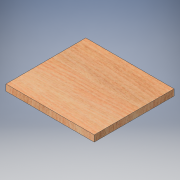
# Autodesk Inventor part: topPlate
Saved by Autodesk Inventor 2016 (Build 200138000, 138)
## iProperties
Created: 2015-09-21
Part Number: topPlate
Material: Generic
Document SubType Name: Modeling
Designer: xdlea
Density: 1 g/cm^3
Appearance: Birch - Natural Polished
Length: 10.500 in
Width: 8.000 in
Thickness: 0.750 in
RailHeight: 2.000 in
Author: xdlea
Autodesk Inventor part; units mm, degrees
ref_plane "YZ Plane" through (0, 0, 0) normal (1, 0, 0) x (0, 1, 0)
ref_plane "XZ Plane" through (0, 0, 0) normal (0, 1, 0) x (-1, 0, 0)
ref_plane "XY Plane" through (0, 0, 0) normal (0, 0, 1) x (1, 0, 0)
sketch "Sketch1" plane through (0, 0, 0) normal (0, 1, 0) x (-1, 0, 0)
  line L0 (133.35, 101.6) -> (-133.35, 101.6)
  line L1 (-133.35, 101.6) -> (-133.35, -101.6)
  line L2 (-133.35, -101.6) -> (133.35, -101.6)
  line L3 (133.35, -101.6) -> (133.35, 101.6)
  line L4 (133.35, 101.6) -> (-133.35, -101.6) construction
  line L5 (-133.35, 101.6) -> (133.35, -101.6) construction
  point P0 (0, 0)
  dimension "d0" = 266.7
  dimension "d1" = 203.2
  constraints: 12 end point, 2 midpoint, 2 parallel, 1 horizontal, 1 perpendicular
  measures "d0" distance of L0.start L0.end
  measures "d1" distance of L0.end L1.end
extrude "Extrusion1" add sketch "Sketch1" along normal blind 19.05
sketch "Sketch2" plane through (-133.35, 0, 101.6) normal (0, 0, 1) x (1, 0, 0)
  line L0 (0, 0) -> (266.7, 0) projected
  line L1 (266.7, 0) -> (266.7, 19.05) projected
  line L2 (0, 19.05) -> (266.7, 19.05) projected
  line L3 (0, 0) -> (0, 19.05) projected
  point P0 (133.35, 0)
extrude "Extrusion2" add sketch "Sketch2" along normal blind 38.1
equation "\"d0\" = Length"
equation "\"d1\" = Width"
equation "\"d2\" = Thickness"
equation "\"d4\" = FrameExtend"
equation "\"Width\" = 203.2"
equation "\"Thickness\" = 19.05"
equation "\"RailHeight\" = 50.8"
equation "\"FrameExtend\" = Thickness_1 + Thickness"
equation "\"Length\" = 266.7"
equation "\"Thickness_1\" = 19.05"
body "Solid1"
